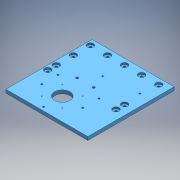
# Autodesk Inventor part: detectionObjHolder
Saved by Autodesk Inventor 2016 (Build 200138000, 138)
## iProperties
Created: 2016-03-08
Part Number: detectionObjHolder
Material: Generic
Document SubType Name: Modeling
Designer: sims01
Density: 1 g/cm^3
Appearance: Default
Author: sims01
Autodesk Inventor part; units mm, degrees
ref_plane "YZ Plane" through (0, 0, 0) normal (1, 0, 0) x (0, 1, 0)
ref_plane "XZ Plane" through (0, 0, 0) normal (0, 1, 0) x (-1, 0, 0)
ref_plane "XY Plane" through (0, 0, 0) normal (0, 0, 1) x (1, 0, 0)
sketch "Sketch1" plane through (0, 0, 0) normal (0, 0, 1) x (1, 0, 0)
  line L0 (-100, 135) -> (140, 135)
  line L1 (140, 135) -> (140, -117.5)
  line L2 (140, -117.5) -> (-100, -117.5)
  line L3 (-100, -117.5) -> (-100, 135)
  point P0 (0, 0)
  dimension "d0" = 240
  dimension "d1" = 140
  dimension "d2" = 252.5
  dimension "d3" = 135
  constraints: 8 end point, 2 parallel, 1 horizontal, 1 perpendicular
  measures "d0" distance of L0.start L0.end
  measures "d1" distance from line of point (0, 0) L1
  measures "d2" distance of L0.end L1.end
  measures "d3" distance from line of point (0, 0) L0
extrude "baseExtrusion" add sketch "Sketch1" along normal blind 10.2
sketch "Sketch2" plane through (0, 0, 10.2) normal (0, 0, 1) x (1, 0, 0)
  circle A0 centre (0, -52.5) radius 22.5
  line L0 (-100, -117.5) -> (140, -117.5) projected
  point P0 (0, 0)
  dimension "d6" = 45
  dimension "d7" = 65
  constraints: 1 centre point, 1 vertical alignment
  measures "d6" diameter of A0
  measures "d7" distance from line of L0 A0.centre
extrude "objectiveExtrusion" cut sketch "Sketch2" against normal through all
sketch "Sketch3" plane through (0, 0, 10.2) normal (0, 0, 1) x (1, 0, 0)
  circle A0 centre (0, -52.5) radius 22.5 projected
  point P0 (0, 0)
  point P1 (-30, -22.5)
  point P2 (30, -22.5)
  point P3 (-30, -82.5)
  point P4 (30, -82.5)
  dimension "d10" = 60
  dimension "d11" = 60
  dimension "d12" = 30
  dimension "d41" = 30
  constraints: 2 horizontal alignment, 2 vertical alignment
  measures "d10" distance of point (30, -22.5) point (-30, -22.5)
  measures "d11" distance of point (30, -82.5) point (30, -22.5)
  measures "d12" horizontal distance of A0.centre point (30, -22.5)
  measures "d41" horizontal distance of A0.centre point (30, -22.5)
hole "60mmCageRodThread" at (-30, -22.5, 10.2) at (30, -22.5, 10.2) at (-30, -82.5, 10.2) at (30, -82.5, 10.2) direction (0, 0, -1) diameter 2.156 end through all thread size "4-40 UNC" class "2B" standard "ANSI Unified Screw Threads"
sketch "Sketch4" plane through (0, 0, 10.2) normal (0, 0, 1) x (1, 0, 0)
  circle A0 centre (0, -52.5) radius 22.5 projected
  line L0 (-100, 135) -> (-100, -117.5) projected
  point P0 (0, 0)
  point P1 (-87.5, 117.5)
  point P2 (112.5, 117.5)
  point P3 (-87.5, 17.5)
  point P4 (112.5, 17.5)
  point P5 (12.5, 117.5)
  point P6 (-37.5, 117.5)
  point P7 (62.5, 117.5)
  point P8 (-87.5, -7.5)
  point P9 (112.5, -7.5)
  point P10 (-87.5, 67.5)
  dimension "d20" = 200
  dimension "d21" = 100
  dimension "d23" = 70
  dimension "d74" = 100
  dimension "d75" = 25
  dimension "d76" = 50
  dimension "d77" = 50
  dimension "d78" = 12.5
  dimension "d79" = 50
  constraints: 7 horizontal alignment, 5 vertical alignment
  measures "d20" distance of point (112.5, 117.5) point (-87.5, 117.5)
  measures "d21" distance of point (-87.5, 17.5) point (-87.5, 117.5)
  measures "d23" vertical distance of A0.centre point (112.5, 17.5)
  measures "d74" distance of point (12.5, 117.5) point (-87.5, 117.5)
  measures "d75" distance of point (-87.5, -7.5) point (-87.5, 17.5)
  measures "d76" distance of point (12.5, 117.5) point (-37.5, 117.5)
  measures "d77" distance of point (12.5, 117.5) point (62.5, 117.5)
  measures "d78" distance from line of L0 point (-87.5, 117.5)
  measures "d79" distance of point (-87.5, 17.5) point (-87.5, 67.5)
hole "m6BreadoardMountingHoles" at (-87.5, 117.5, 10.2) at (112.5, 117.5, 10.2) at (-87.5, 17.5, 10.2) at (112.5, 17.5, 10.2) at (12.5, 117.5, 10.2) at (-87.5, -7.5, 10.2) at (112.5, -7.5, 10.2) at (62.5, 117.5, 10.2) at (-37.5, 117.5, 10.2) at (-87.5, 67.5, 10.2) direction (0, 0, -1) diameter 6.6 end through all counterbore diameter 18 counterbore depth 4.8 clearance for "Hex Head Cap Screw ISO 24017" size "M6" standard "ISO"
sketch "Sketch5" plane through (0, 0, 0) normal (0, 0, -1) x (-1, 0, 0)
  circle A0 centre (0, -52.5) radius 22.5 projected
  point P0 (0, 0)
  point P1 (-8.4, 57.5)
  point P2 (-107.3, 67.7)
  dimension "d31" = 110
  dimension "d40" = 8.4
  dimension "d72" = 98.9
  dimension "d73" = 10.2
  measures "d31" vertical distance of A0.centre point (-8.4, 57.5)
  measures "d40" horizontal distance of point (0, 0) point (-8.4, 57.5)
  measures "d72" horizontal distance of point (-8.4, 57.5) point (-107.3, 67.7)
  measures "d73" vertical distance of point (-8.4, 57.5) point (-107.3, 67.7)
hole "m4MirrorTLMountingHoles" at (8.4, 57.5, 0) at (107.3, 67.7, 0) direction (0, 0, 1) diameter 4.5 end through all counterbore diameter 13 counterbore depth 3.4 clearance for "Hex Head Cap Screw ISO 24017" size "M4" standard "ISO"
sketch "Sketch6" plane through (0, 0, 10.2) normal (0, 0, 1) x (1, 0, 0)
  circle A0 centre (-30, -22.5) radius 1.078 projected
  point P0 (0, 0)
  point P1 (-60, -5)
  point P2 (60, -5)
  point P3 (-60, -52.5)
  point P4 (60, -52.5)
  point P5 (0, -107.5)
  dimension "d42" = 120
  dimension "d43" = 60
  dimension "d44" = 47.5
  dimension "d45" = 55
  dimension "d46" = 30
  constraints: 3 vertical alignment, 2 horizontal alignment
  measures "d42" distance of point (60, -5) point (-60, -5)
  measures "d43" horizontal distance of point (60, -5) point (0, 0)
  measures "d44" distance of point (-60, -52.5) point (-60, -5)
  measures "d45" vertical distance of point (0, -107.5) point (-60, -52.5)
  measures "d46" horizontal distance of point (-60, -52.5) A0.centre
hole "m6objectiveHolderMountingHoles" at (-60, -5, 10.2) at (60, -5, 10.2) at (-60, -52.5, 10.2) at (60, -52.5, 10.2) at (0, -107.5, 10.2) direction (0, 0, -1) diameter 4.917 end through all thread size "M6x1" class "6H" standard "ISO Metric profile"
sketch "Sketch7" plane through (0, 0, 0) normal (0, 0, -1) x (-1, 0, 0)
  circle A0 centre (0, -52.5) radius 22.5 projected
  point P0 (0, 0)
  point P1 (-24.25, 15.5)
  point P2 (24.25, 15.5)
  dimension "d54" = 48.5
  dimension "d55" = 24.25
  dimension "d56" = 68
  constraints: 1 horizontal alignment
  measures "d54" distance of point (24.25, 15.5) point (-24.25, 15.5)
  measures "d55" horizontal distance of point (0, 0) point (-24.25, 15.5)
  measures "d56" vertical distance of A0.centre point (-24.25, 15.5)
hole "filterwheelMountingHoles" at (24.25, 15.5, 0) at (-24.25, 15.5, 0) direction (0, 0, 1) diameter 6.6 depth 17.1 tip angle 118 counterbore diameter 10 counterbore depth 4.8 clearance for "Hex Head Cap Screw ISO 24017" size "M6" standard "ISO"
equation "\"d12\" = 0.5 * d11"
equation "\"d74\" = 0.5 * d20"
equation "\"d76\" = 0.5 * d74"
equation "\"d77\" = d76"
equation "\"d79\" = 0.5 * d21"
equation "\"d43\" = 0.5 * d42"
equation "\"d55\" = 0.5 * d54"
body "Solid1"
